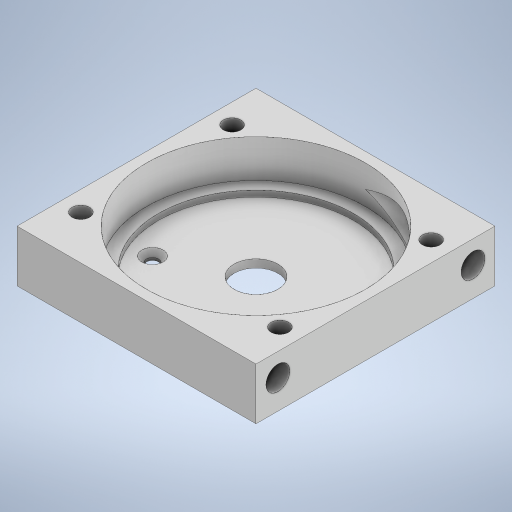
# Autodesk Inventor part: Base
Saved by Autodesk Inventor 2023 (Build 270158000, 158)
## iProperties
Created: 2023-04-01
Part Number: Base
Material: Genérico
Document SubType Name: Modeling
Designer: sergi
Density: 1 g/cm^3
Appearance: Valor por defecto
Author: sergi
Autodesk Inventor part; units mm, degrees
ref_plane "YZ Plane" through (0, 0, 0) normal (1, 0, 0) x (0, 1, 0)
ref_plane "XZ Plane" through (0, 0, 0) normal (0, 1, 0) x (-1, 0, 0)
ref_plane "XY Plane" through (0, 0, 0) normal (0, 0, 1) x (1, 0, 0)
sketch "Boceto1" plane through (0, 0, 0) normal (0, 1, 0) x (-1, 0, 0)
  line L0 (-30, -30) -> (30, -30)
  line L1 (30, -30) -> (30, 30)
  line L2 (30, 30) -> (-30, 30)
  line L3 (-30, 30) -> (-30, -30)
  line L4 (-30, -30) -> (30, 30) construction
  line L5 (30, -30) -> (-30, 30) construction
  point P0 (0, 0)
  dimension "d0" = 60
  dimension "d1" = 60
  constraints: 12 end point, 2 midpoint, 2 parallel, 1 horizontal, 1 perpendicular
  measures "d0" distance of L2.end L1.end
  measures "d1" distance of L1.end L0.end
extrude "Extrusión1" add sketch "Boceto1" along normal blind 13
sketch "Boceto2" plane through (0, 13, 0) normal (0, 1, 0) x (1, 0, 0)
  circle A0 centre (0, 0) radius 27.5
  dimension "d4" = 55
  constraints: 1 centre point, 1 coincident
  measures "d4" diameter of A0
extrude "Extrusión2" cut sketch "Boceto2" against normal blind 11
sketch "Boceto3" plane through (0, 2, 0) normal (0, 1, 0) x (1, 0, 0)
  circle A0 centre (0, 0) radius 27.5 projected
  constraints: 1 coincident
hole "Agujero1" at (0, 2, 0) direction (0, -1, 0) diameter 11 depth 2
sketch "Boceto4" plane through (0, 13, 0) normal (0, 1, 0) x (1, 0, 0)
  line L0 (-30, -30) -> (30, -30) projected
  line L1 (30, -30) -> (30, 30) projected
  point P0 (0, 0)
  point P1 (25, -19)
  dimension "d14" = 11
  dimension "d15" = 5
  measures "d14" distance from line of L0 point (25, -19)
  measures "d15" distance from line of L1 point (25, -19)
hole "Agujero2" at (25, 13, 19) direction (0, -1, 0) diameter 4.4 end through all
pattern_linear "Patrón rectangular1" count 2 spacing 38 along (0, 0, -1) count 2 spacing 50 along (-1, 0, 0) of "Agujero2"
sketch "Boceto5" plane through (0, 2, 0) normal (0, 1, 0) x (1, 0, 0)
  circle A0 centre (0, 0) radius 24.5
  circle A1 centre (0, 0) radius 27.5
  dimension "d29" = 49
  dimension "d30" = 55
  constraints: 2 centre point, 2 coincident
  measures "d29" diameter of A0
  measures "d30" diameter of A1
extrude "Extrusión3" add sketch "Boceto5" along normal blind 1.5
sketch "Boceto6" plane through (30, 0, 30) normal (1, 0, 0) x (0, 0, -1)
  line L0 (2.5, 13) -> (57.5, 13) projected
  line L1 (2.5, 13) -> (2.5, 3.5) projected
  line L2 (2.5, 3.5) -> (57.5, 3.5) projected
  line L3 (57.5, 13) -> (57.5, 3.5) projected
  line L4 (2.5, 13) -> (2.5, 11)
  line L5 (2.5, 11) -> (57.5, 11)
  line L6 (5.5, 3.5) -> (54.5, 3.5) projected
  line L7 (5.5, 3.5) -> (5.5, 11)
  circle A0 centre (5.5, 7.25) radius 3
  circle A1 centre (54.5, 7.25) radius 3
  point P0 (30, 0)
  point P1 (5.5, 7.25)
  dimension "d49" = 2
  dimension "d50" = 6
  dimension "d51" = 6
  constraints: 6 end point, 3 point on line, 2 centre point, 2 coincident, 2 perpendicular, 1 midpoint
  measures "d49" distance of L1.start L4.end
  measures "d50" diameter of A0
  measures "d51" diameter of A1
hole "Agujero3" at (30, 7.25, 24.5) at (30, 7.25, -24.5) direction (-1, 0, 0) diameter 6 depth 30
sketch "Boceto7" plane through (0, 2, 0) normal (0, 1, 0) x (1, 0, 0)
  circle A0 centre (-17.4927, -8.5006) radius 1.9922 projected
  circle A1 centre (17.4936, -8.4925) radius 2.0099 projected
  point P0 (0, 0)
hole "Agujero4" at (17.4936, 2, 8.4925) at (-17.4927, 2, 8.5006) direction (0, -1, 0) diameter 3 end through all countersink diameter 5.3 countersink angle 80
